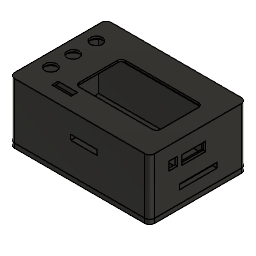
带螺丝的照相机外壳 (Autodesk Fusion 360 design; units mm, degrees)
part number: 2026-01-23-16-43-48-473
Autodesk Fusion 360 part; units mm, degrees
sketch "草图1" plane through (0, 0, 0) normal (0, 0, 1) x (1, 0, 0)
  line L0 (0, 0) -> (56, 0)
  line L1 (56, 0) -> (56, -32.7)
  line L2 (56, -32.7) -> (0, -32.7)
  line L3 (0, -32.7) -> (0, 0)
  dimension "d1" = 56
  dimension "d2" = 32.7
  constraint horizontal L0
  constraint vertical L1
  constraint horizontal L2
  constraint vertical L3
  constraint coincident L0.start L3.end
  measures "d1" distance of L0.start L0.end
  measures "d2" distance of L0.start L2.end
extrude "盒子主体" add sketch "草图1" along normal blind 24.1 makes body 1
shell "盒子抽壳" thickness 1.8 removed faces 0 bodies 1
extrude "前壁加厚" add 1 faces at (37.3333, -32.7, 8.0333) along direction (0, -1, 0) blind 3 on bodies 1 bodies 1
extrude "后壁加厚" add 1 faces at (18.6667, 0, 8.0333) along direction (0, 1, 0) blind 3 on bodies 1 bodies 1
sketch "草图2" plane through (0, 0, 24.1) normal (0, 0, 1) x (-1, 0, 0)
  line L0 (-56, 35.7) -> (-56, -3)
  line L1 (-56, -3) -> (0, -3)
  line L2 (0, -3) -> (0, 35.7)
  line L3 (0, 35.7) -> (-56, 35.7)
  line L4 (-21, -3) -> (-21, 6.164) construction
  line L5 (-6.433, 6.164) -> (-7.239, 6.164) construction
  line L6 (-7.239, 6.164) -> (-7.239, 6.97) construction
  line L7 (0, -3) -> (-56, 35.7) construction
  line L8 (0, 35.7) -> (-56, -3) construction
  circle A0 centre (-5.43, 6.36) radius 2.35
  circle A1 centre (-5.43, 15.64) radius 2.35
  circle A2 centre (-5.43, 24.55) radius 2.35
  line L9 (-19.4435, 30.465) -> (-19.4435, 27.962)
  line L10 (-19.4435, 27.962) -> (-11.7695, 27.962)
  line L11 (-11.7695, 30.465) -> (-19.4435, 30.465)
  line L12 (-11.7695, 27.962) -> (-11.7695, 30.465)
  line L13 (-56, 35.7) -> (-56, 26.536) construction
  line L14 (-56, 26.536) -> (-49.567, 26.536) construction
  line L15 (-49.567, 26.536) -> (-12.067, 26.536)
  line L16 (-12.067, 26.536) -> (-12.067, 6.536)
  line L17 (-12.067, 6.536) -> (-49.567, 6.536)
  line L18 (-49.567, 6.536) -> (-49.567, 26.536)
  line L19 (-49.567, 26.536) -> (-48.761, 26.536) construction
  line L20 (-48.761, 26.536) -> (-48.761, 25.73) construction
  line L21 (-48.761, 25.73) -> (-16.361, 25.73)
  line L22 (-16.361, 25.73) -> (-16.361, 7.33)
  line L23 (-16.361, 7.33) -> (-48.761, 7.33)
  line L24 (-48.761, 7.33) -> (-48.761, 25.73)
  dimension "d78" = 9.164
  dimension "d79" = 6.433
  dimension "d80" = 37.5
  dimension "d81" = 20
  dimension "d82" = 0.806
  dimension "d83" = 0.806
  dimension "d84" = 32.4
  dimension "d85" = 18.4
  constraint coincident L1 L4.start
  constraint perpendicular L1 L4
  constraint perpendicular L5 L6
  constraint coincident L1.end L2.start
  constraint coincident L0.start L3.end
  constraint coincident L2.end L3.start
  constraint coincident L0.end L1.start
  constraint perpendicular L3 L13
  constraint perpendicular L13 L14
  constraint horizontal L15
  constraint vertical L16
  constraint horizontal L17
  constraint vertical L18
  constraint perpendicular L18 L19
  constraint perpendicular L19 L20
  constraint horizontal L21
  constraint vertical L22
  constraint horizontal L23
  constraint vertical L24
  measures "d78" distance of L0.start L13.end
  measures "d79" distance of L13.end L14.end
  measures "d80" distance of L14.end L15.end
  measures "d81" distance of L14.end L17.end
  measures "d82" distance of L14.end L19.end
  measures "d83" distance of L19.end L20.end
  measures "d84" distance of L20.end L21.end
  measures "d85" distance of L20.end L23.end
sketch "草图3" plane through (56, 0, 0) normal (1, 0, 0) x (0, 1, 0)
  line L0 (-35.7, 0) -> (3, 0)
  line L1 (3, 0) -> (3, 24.1)
  line L2 (3, 24.1) -> (-35.7, 24.1)
  line L3 (-35.7, 24.1) -> (-35.7, 0)
  line L4 (-35.7, 24.1) -> (-35.7, 18.648) construction
  line L5 (-35.7, 24.1) -> (-35.7, 18.266) construction
  line L6 (-35.7, 18.648) -> (-27.995, 18.648) construction
  line L7 (-35.7, 18.266) -> (-22.859, 18.266) construction
  line L8 (-27.995, 18.648) -> (-24.595, 18.648)
  line L9 (-24.595, 18.648) -> (-24.595, 15.248)
  line L10 (-24.595, 15.248) -> (-27.995, 15.248)
  line L11 (-27.995, 15.248) -> (-27.995, 18.648)
  line L12 (-22.859, 18.266) -> (-13.359, 18.266)
  line L13 (-13.359, 18.266) -> (-13.359, 14.666)
  line L14 (-13.359, 14.666) -> (-22.859, 14.666)
  line L15 (-22.859, 14.666) -> (-22.859, 18.266)
  line L16 (-35.7, 24.1) -> (-35.7, 8.684) construction
  line L17 (-35.7, 8.684) -> (-23.839, 8.684) construction
  line L18 (-23.839, 8.684) -> (-8.839, 8.684)
  line L19 (-8.839, 8.684) -> (-8.839, 6.684)
  line L20 (-8.839, 6.684) -> (-23.839, 6.684)
  line L21 (-23.839, 6.684) -> (-23.839, 8.684)
  dimension "d29" = 5.452
  dimension "d30" = 5.834
  dimension "d31" = 7.705
  dimension "d32" = 12.841
  dimension "d33" = 3.4
  dimension "d34" = 3.4
  dimension "d35" = 9.5
  dimension "d36" = 3.6
  dimension "d37" = 15.416
  dimension "d38" = 11.861
  dimension "d39" = 15
  dimension "d40" = 2
  constraint coincident L2.end L3.start
  constraint perpendicular L2 L4
  constraint perpendicular L2 L5
  constraint perpendicular L3 L6
  constraint perpendicular L5 L7
  constraint horizontal L8
  constraint vertical L9
  constraint horizontal L10
  constraint vertical L11
  constraint horizontal L12
  constraint vertical L13
  constraint horizontal L14
  constraint vertical L15
  constraint parallel L3 L16
  constraint perpendicular L16 L17
  constraint horizontal L18
  constraint vertical L19
  constraint horizontal L20
  constraint vertical L21
  measures "d29" distance of L2.end L4.end
  measures "d30" distance of L2.end L5.end
  measures "d31" distance of L4.end L6.end
  measures "d32" distance of L5.end L7.end
  measures "d33" distance of L6.end L8.end
  measures "d34" distance of L6.end L10.end
  measures "d35" distance of L7.end L12.end
  measures "d36" distance of L7.end L14.end
  measures "d37" distance of L2.end L16.end
  measures "d38" distance of L16.end L17.end
  measures "d39" distance of L17.end L18.end
  measures "d40" distance of L17.end L20.end
sketch "草图4" plane through (0, -35.7, 0) normal (0, -1, 0) x (1, 0, 0)
  line L0 (0, 0) -> (56, 0)
  line L1 (56, 0) -> (56, 24.1)
  line L2 (56, 24.1) -> (0, 24.1)
  line L3 (0, 24.1) -> (0, 0)
  line L4 (0, 24.1) -> (0, 16) construction
  line L5 (0, 16) -> (24.5, 16) construction
  line L6 (24.5, 16) -> (35, 16)
  line L7 (35, 16) -> (35, 14)
  line L8 (35, 14) -> (24.5, 14)
  line L9 (24.5, 14) -> (24.5, 16)
  dimension "d41" = 8.1
  dimension "d42" = 24.5
  dimension "d43" = 10.5
  dimension "d44" = 2
  constraint coincident L2.end L3.start
  constraint perpendicular L2 L4
  constraint perpendicular L3 L5
  constraint horizontal L6
  constraint vertical L7
  constraint horizontal L8
  constraint vertical L9
  measures "d41" distance of L2.end L4.end
  measures "d42" distance of L4.end L5.end
  measures "d43" distance of L5.end L6.end
  measures "d44" distance of L5.end L8.end
ref_plane "工作平面1" through (28, -16.35, 1.8) normal (0, 0, -1) x (-1, 0, 0)
split "分割1" by plane through (28, -16.35, 1.8) normal (0, 0, -1) bodies 1 makes body 2 at (18.6667, -22.8, 0)
sketch "草图5" plane through (0, 0, 1.8) normal (0, 0, -1) x (1, 0, 0)
  line L0 (56, 35.7) -> (0, 35.7)
  line L1 (0, 35.7) -> (0, -3)
  line L2 (0, -3) -> (56, -3)
  line L3 (56, -3) -> (56, 35.7)
  line L4 (1.8, 1.8) -> (1.8, 30.9)
  line L5 (1.8, 30.9) -> (54.2, 30.9)
  line L6 (54.2, 30.9) -> (54.2, 1.8)
  line L7 (54.2, 1.8) -> (1.8, 1.8)
  circle A0 centre (3.3512, 33.3474) radius 0.9
  circle A1 centre (3.3512, 33.3474) radius 1.75
  line L8 (0, 35.7) -> (56, -3) construction
  line L9 (0, -3) -> (56, 35.7) construction
  line L10 (28, 16.35) -> (0, 16.35) construction
  line L11 (28, 16.35) -> (28, -3) construction
  circle A2 centre (3.3512, -0.6474) radius 1.75
  circle A3 centre (3.3512, -0.6474) radius 0.9
  circle A4 centre (52.6488, 33.3474) radius 1.75
  circle A5 centre (52.6488, 33.3474) radius 0.9
  circle A6 centre (52.6488, -0.6474) radius 0.9
  circle A7 centre (52.6488, -0.6474) radius 1.75
  dimension "d46" = 1.8
  dimension "d47" = 3.5
  constraint concentric A0 A1
  constraint coincident L0.end L1.start
  constraint coincident L2.end L3.start
  constraint coincident L1.end L2.start
  constraint coincident L0.start L3.end
  constraint midpoint L9 L10.start
  constraint perpendicular L4 L10
  constraint midpoint L2 L11.end
  constraint symmetric A0 L10 A3
  constraint symmetric A1 L10 A2
  constraint symmetric A0 L11 A5
  constraint symmetric A1 L11 A4
  constraint symmetric L11 A2 A7
  constraint symmetric L11 A3 A6
  measures "d46" diameter of A0
  measures "d47" diameter of A1
extrude "拉伸4" cut sketch "草图5" against normal blind 4 contours A0 | A3 | A5 | A6 bodies 1
sketch "草图6" plane through (0, 0, 0) normal (0, 0, -1) x (1, 0, 0)
  line L0 (0, 35.7) -> (0, -3)
  line L1 (0, -3) -> (56, -3)
  line L2 (56, -3) -> (56, 35.7)
  line L3 (56, 35.7) -> (0, 35.7)
  circle A0 centre (3.3512, 33.3474) radius 1.75
  circle A1 centre (52.6488, 33.3474) radius 1.75
  circle A2 centre (52.6488, -0.6474) radius 1.75
  circle A3 centre (3.3512, -0.6474) radius 1.75
  circle A4 centre (52.6488, -0.6474) radius 0.9
  circle A5 centre (3.3512, -0.6474) radius 0.9
  circle A6 centre (3.3512, 33.3474) radius 0.9
  circle A7 centre (52.6488, 33.3474) radius 0.9
  line L4 (56, 35.7) -> (56, 20.95) construction
  line L5 (56, 20.95) -> (46, 20.95) construction
  line L6 (46, 20.95) -> (36.8, 20.95)
  line L7 (36.8, 20.95) -> (36.8, 11.75)
  line L8 (36.8, 11.75) -> (46, 11.75)
  line L9 (46, 11.75) -> (46, 20.95)
  line L10 (46, 11.75) -> (36.8, 20.95) construction
  line L11 (46, 20.95) -> (36.8, 11.75) construction
  circle A8 centre (41.4, 16.35) radius 4
  circle A9 centre (41.4, 16.35) radius 8.2057
  dimension "d70" = 14.75
  dimension "d71" = 10
  dimension "d72" = 9.2
  dimension "d73" = 9.2
  dimension "d128" = 8
  constraint coincident L2.end L3.start
  constraint perpendicular L3 L4
  constraint perpendicular L4 L5
  constraint horizontal L6
  constraint vertical L7
  constraint horizontal L8
  constraint vertical L9
  constraint midpoint L11 A8.centre
  constraint concentric A8 A9
  measures "d70" distance of L2.end L4.end
  measures "d71" distance of L4.end L5.end
  measures "d72" distance of L5.end L6.end
  measures "d73" distance of L5.end L8.end
  measures "d128" diameter of A8
extrude "拉伸5" cut sketch "草图6" against normal blind 1.2 contours A0 | A1 | A2 | A3 | A4 | A5 | A6 | A7 bodies 2
extrude "拉伸6" cut sketch "草图6" against normal blind 1.8 contours A4 | A5 | A6 | A7 bodies 2
extrude "拉伸7" cut sketch "草图4" against normal blind 4.8 contours L6 L7 L8 L9 bodies 1
extrude "拉伸9" cut sketch "草图3" against normal blind 1.8 contours L8 L9 L10 L11 | L12 L13 L14 L15 | L18 L19 L20 L21 bodies 1
fillet "圆角3" radius 2 8 edges at (56, 3, 12.95) (56, -35.7, 12.95) (0, 3, 12.95) (0, -35.7, 12.95) (56, 3, 0.9) (56, -35.7, 0.9) (0, 3, 0.9) (0, -35.7, 0.9) on bodies 1 2
extrude "拉伸12" cut sketch "草图6" against normal blind 1.8 contours L6 L7 L8 L9 | A8 bodies 2
extrude "拉伸13" cut sketch "草图2" against normal blind 1.8 contours A0 | A1 | A2 | L9 L10 L11 L12 bodies 1
extrude "拉伸14" cut sketch "草图2" against normal blind 1.8 contours L21 L22 L23 L24 bodies 1
sketch "草图8" plane through (0, 0, 22.3) normal (0, 0, -1) x (1, 0, 0)
  line L0 (16.361, 7.33) -> (16.361, 25.73)
  line L1 (16.361, 25.73) -> (48.761, 25.73)
  line L2 (48.761, 25.73) -> (48.761, 7.33)
  line L3 (48.761, 7.33) -> (16.361, 7.33)
  circle A0 centre (5.43, 24.55) radius 2.35
  circle A1 centre (5.43, 15.64) radius 2.35
  line L4 (11.7695, 30.465) -> (19.4435, 30.465)
  line L5 (19.4435, 30.465) -> (19.4435, 27.962)
  line L6 (19.4435, 27.962) -> (11.7695, 27.962)
  line L7 (11.7695, 27.962) -> (11.7695, 30.465)
  circle A2 centre (5.43, 6.36) radius 2.35
  line L8 (54.2, 30.9) -> (1.8, 30.9)
  line L9 (1.8, 30.9) -> (1.8, 1.8)
  line L10 (1.8, 1.8) -> (54.2, 1.8)
  line L11 (54.2, 1.8) -> (54.2, 30.9)
  line L12 (49.567, 6.536) -> (49.567, 26.536)
  line L13 (12.067, 6.536) -> (49.567, 6.536)
  line L14 (12.067, 26.536) -> (12.067, 6.536)
  line L15 (49.567, 26.536) -> (12.067, 26.536)
extrude "拉伸15" cut sketch "草图8" against normal blind 1 contours L12 L13 L14 L15 bodies 1
fillet "圆角4" radius 1.5 4 edges at (49.567, -6.536, 22.8) (49.567, -26.536, 22.8) (12.067, -26.536, 22.8) (12.067, -6.536, 22.8) on bodies 1
fillet "圆角5" radius 1.5 4 edges at (48.761, -25.73, 23.7) (48.761, -7.33, 23.7) (16.361, -7.33, 23.7) (16.361, -25.73, 23.7) on bodies 1
ref_plane "工作平面2" through (28, -16.35, 25.1) normal (0, 0, 1) x (1, 0, 0)
sketch "草图9" plane through (0, 0, 25.1) normal (0, 0, 1) x (1, 0, 0)
  line L0 (19.4435, -30.465) -> (11.7695, -30.465)
  line L1 (19.4435, -27.962) -> (19.4435, -30.465)
  line L2 (11.7695, -27.962) -> (19.4435, -27.962)
  line L3 (11.7695, -30.465) -> (11.7695, -27.962)
  line L4 (19.2435, -28.162) -> (19.2435, -30.265)
  line L5 (19.2435, -30.265) -> (11.9695, -30.265)
  line L6 (11.9695, -30.265) -> (11.9695, -28.162)
  line L7 (11.9695, -28.162) -> (19.2435, -28.162)
  line L8 (11.9695, -30.265) -> (8.9695, -30.265)
  line L9 (8.9695, -30.265) -> (8.9695, -28.162)
  line L10 (8.9695, -28.162) -> (11.9695, -28.162)
  line L11 (11.9695, -28.162) -> (11.9695, -30.265)
  line L12 (19.2435, -30.265) -> (22.2435, -30.265)
  line L13 (22.2435, -30.265) -> (22.2435, -28.162)
  line L14 (22.2435, -28.162) -> (19.2435, -28.162)
  line L15 (19.2435, -28.162) -> (19.2435, -30.265)
  circle A0 centre (5.43, -24.55) radius 2.35
  circle A1 centre (5.43, -15.64) radius 2.35
  circle A2 centre (5.43, -6.36) radius 2.35
  circle A3 centre (5.43, -24.55) radius 2.15
  circle A4 centre (5.43, -24.55) radius 3.15
  dimension "d95" = 0.2
  dimension "d96" = 3
  dimension "d97" = 3
  dimension "d104" = -0.2
  dimension "d105" = 1
  constraint horizontal L8
  constraint vertical L9
  constraint horizontal L10
  constraint vertical L11
  constraint horizontal L12
  constraint vertical L13
  constraint horizontal L14
  constraint vertical L15
  measures "d96" distance of L5.end L8.end
  measures "d97" distance of L4.end L12.end
extrude "拉伸16" add sketch "草图9" along normal blind 0.5 separate body contours L1 L4 L12 L14 L15 | L1 L12 L13 L14 | L3 L8 L9 L10 | L3 L6 L8 L10 L11 | A0 | A4 makes body 3 at (10.9695, -28.863, 25.1) makes body 4 at (21.2435, -29.564, 25.1) makes body 5 at (8.2269, -24.8133, 25.1)
extrude "拉伸17" add sketch "草图9" along normal blind 4.5 contours L4 L5 L6 L7 L11 L15 | A3 bodies 3 5 4
fillet "圆角6" radius 0.5 4 edges at (11.9695, -28.162, 27.6) (11.9695, -30.265, 27.6) (19.2435, -28.162, 27.6) (19.2435, -30.265, 27.6) on bodies 3
ref_plane "工作平面3" through (57, -16.35, 12.95) normal (1, 0, 0) x (0, 1, 0)
sketch "草图10" plane through (57, 0, 0) normal (1, 0, 0) x (0, 1, 0)
  line L0 (-27.995, 15.248) -> (-27.995, 18.648)
  line L1 (-27.995, 18.648) -> (-24.595, 18.648)
  line L2 (-24.595, 18.648) -> (-24.595, 15.248)
  line L3 (-24.595, 15.248) -> (-27.995, 15.248)
  line L4 (-27.795, 15.448) -> (-27.795, 18.448)
  line L5 (-27.795, 18.448) -> (-24.795, 18.448)
  line L6 (-24.795, 18.448) -> (-24.795, 15.448)
  line L7 (-24.795, 15.448) -> (-27.795, 15.448)
  line L8 (-23.795, 14.448) -> (-28.795, 14.448)
  line L9 (-28.795, 14.448) -> (-28.795, 19.448)
  line L10 (-28.795, 19.448) -> (-23.795, 19.448)
  line L11 (-23.795, 19.448) -> (-23.795, 14.448)
  dimension "d107" = 0.2
  dimension "d108" = -1
extrude "拉伸18" add sketch "草图10" along normal blind 0.5 separate body contours L0 L1 L2 L3 | L8 L9 L10 L11 makes body 6
extrude "拉伸19" add sketch "草图10" along normal blind 5 contours L4 L5 L6 L7 bodies 6
fillet "圆角7" radius 0.5 4 edges at (59.75, -27.795, 18.448) (59.75, -24.795, 15.448) (59.75, -24.795, 18.448) (59.75, -27.795, 15.448) on bodies 6
sketch "草图11" plane through (54.2, 0, 0) normal (-1, 0, 0) x (0, -1, 0)
  line L0 (24.595, 15.248) -> (24.595, 18.648)
  line L1 (24.595, 18.648) -> (27.995, 18.648)
  line L2 (27.995, 18.648) -> (27.995, 15.248)
  line L3 (27.995, 15.248) -> (24.595, 15.248)
  line L4 (13.359, 14.666) -> (13.359, 18.266)
  line L5 (13.359, 18.266) -> (22.859, 18.266)
  line L6 (22.859, 18.266) -> (22.859, 14.666)
  line L7 (22.859, 14.666) -> (13.359, 14.666)
  line L8 (8.839, 6.684) -> (8.839, 8.684)
  line L9 (8.839, 8.684) -> (23.839, 8.684)
  line L10 (23.839, 8.684) -> (23.839, 6.684)
  line L11 (23.839, 6.684) -> (8.839, 6.684)
  line L12 (1.8, 1.8) -> (30.9, 1.8)
  line L13 (30.9, 1.8) -> (30.9, 22.3)
  line L14 (30.9, 22.3) -> (1.8, 22.3)
  line L15 (1.8, 22.3) -> (1.8, 1.8)
  line L16 (23.795, 19.448) -> (23.795, 14.448)
  line L17 (23.795, 14.448) -> (28.795, 14.448)
  line L18 (28.795, 14.448) -> (28.795, 19.448)
  line L19 (28.795, 19.448) -> (23.795, 19.448)
  line L20 (23.595, 19.648) -> (23.595, 14.248)
  line L21 (23.595, 14.248) -> (28.995, 14.248)
  line L22 (28.995, 14.248) -> (28.995, 19.648)
  line L23 (28.995, 19.648) -> (23.595, 19.648)
  line L24 (22.859, 14.666) -> (13.359, 14.666)
  line L25 (22.859, 18.266) -> (22.859, 14.666)
  line L26 (13.359, 18.266) -> (22.859, 18.266)
  line L27 (13.359, 14.666) -> (13.359, 18.266)
  line L28 (13.159, 18.466) -> (23.059, 18.466)
  line L29 (23.059, 18.466) -> (23.059, 14.466)
  line L30 (23.059, 14.466) -> (13.159, 14.466)
  line L31 (13.159, 14.466) -> (13.159, 18.466)
  dimension "d115" = 0.2
  dimension "d116" = -0.2
extrude "拉伸20" cut sketch "草图11" against normal blind 0.8 contours L16 L17 L18 L19 | L20 L21 L22 L23 | L28 L29 L30 L31 bodies 1
sketch "草图12" plane through (0, 0, 22.3) normal (0, 0, -1) x (1, 0, 0)
  line L0 (12.067, 8.036) -> (12.067, 25.036)
  arc A0 (13.567, 26.536) -> (12.067, 25.036) centre (13.567, 25.036) ccw
  line L1 (13.567, 26.536) -> (48.067, 26.536)
  arc A1 (49.567, 25.036) -> (48.067, 26.536) centre (48.067, 25.036) ccw
  line L2 (49.567, 25.036) -> (49.567, 8.036)
  arc A2 (48.067, 6.536) -> (49.567, 8.036) centre (48.067, 8.036) ccw
  line L3 (48.067, 6.536) -> (13.567, 6.536)
  arc A3 (12.067, 8.036) -> (13.567, 6.536) centre (13.567, 8.036) ccw
  circle A4 centre (5.43, 24.55) radius 2.35
  circle A5 centre (5.43, 15.64) radius 2.35
  line L4 (11.7695, 30.465) -> (19.4435, 30.465)
  line L5 (19.4435, 30.465) -> (19.4435, 27.962)
  line L6 (19.4435, 27.962) -> (11.7695, 27.962)
  line L7 (11.7695, 27.962) -> (11.7695, 30.465)
  circle A6 centre (5.43, 6.36) radius 2.35
  line L8 (54.2, 30.9) -> (1.8, 30.9)
  line L9 (1.8, 30.9) -> (1.8, 1.8)
  line L10 (1.8, 1.8) -> (54.2, 1.8)
  line L11 (54.2, 1.8) -> (54.2, 30.9)
  circle A7 centre (5.43, 24.55) radius 3.15
  line L12 (11.9695, 30.265) -> (8.9695, 30.265)
  line L13 (8.9695, 30.265) -> (8.9695, 28.162)
  line L14 (8.9695, 28.162) -> (11.9695, 28.162)
  line L15 (19.2435, 30.265) -> (11.9695, 30.265)
  line L16 (11.9695, 28.162) -> (19.2435, 28.162)
  line L17 (19.2435, 30.265) -> (22.2435, 30.265)
  line L18 (22.2435, 28.162) -> (19.2435, 28.162)
  line L19 (22.2435, 30.265) -> (22.2435, 28.162)
  circle A8 centre (5.43, 15.64) radius 3.15
  circle A9 centre (5.43, 6.36) radius 3.15
  circle A10 centre (5.43, 24.55) radius 3.35
  circle A11 centre (5.43, 15.64) radius 3.35
  line L20 (11.9695, 27.962) -> (19.2435, 27.962)
  line L21 (22.4435, 27.962) -> (19.2435, 27.962)
  line L22 (22.4435, 30.465) -> (22.4435, 27.962)
  line L23 (19.2435, 30.465) -> (22.4435, 30.465)
  line L24 (19.2435, 30.465) -> (11.9695, 30.465)
  line L25 (11.9695, 30.465) -> (8.7695, 30.465)
  line L26 (8.7695, 30.465) -> (8.7695, 27.962)
  line L27 (8.7695, 27.962) -> (11.9695, 27.962)
  circle A12 centre (5.43, 6.36) radius 3.35
  dimension "d119" = 6.3
  dimension "d120" = 6.3
  dimension "d121" = 0.2
  dimension "d122" = 0.2
  dimension "d124" = 0.2
  dimension "d125" = 0.2
  constraint concentric A5 A8
  constraint concentric A6 A9
  measures "d119" diameter of A8
  measures "d120" diameter of A9
extrude "拉伸21" cut sketch "草图12" against normal blind 1 contours L7 L12 L13 L14 L25 L26 L27 | L7 L12 L13 L14 | L5 L17 L18 L19 L21 L22 L23 | L5 L17 L18 L19 | A7 | A8 | A9 | A10 | A11 | A12 bodies 1
extrude "拉伸22" add sketch "草图6" along normal blind 3.5 contours L6 L7 L8 L9 | A9 bodies 2
chamfer "倒角1" distance 1.5 angle 45 1 edges at (37.6707, -17.7965, -3.5) on bodies 2
hidden bodies 3 5 6
equation "d31 = 4.705 mm + 3 mm"
equation "d32 = 9.841 mm + 3 mm"
equation "d38 = 8.861 mm + 3 mm"
equation "d41 = 5.1 mm + 3 mm"
equation "d70 = 11.75 mm + 3 mm"
equation "d78 = 6.164 mm + 3 mm"
named bodies: "主体", "底盖", "快门按键", "功能按键", "电源开关"
